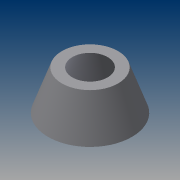
# Autodesk Inventor part: pin
Saved by Autodesk Inventor 2020 (Build 240168000, 168)
## iProperties
Created: 2021-10-08
Part Number: pin
Material: Genérico
Document SubType Name: Modeling
Designer: MATT
Density: 1 g/cm^3
Appearance: Por defecto
Mass: 0.101116 g
Surface Area: 8.28121 cm^2
Volume: 0.101116 cm^3
Author: MATT
Autodesk Inventor part; units mm, degrees
ref_plane "YZ Plane" through (0, 0, 0) normal (1, 0, 0) x (0, 1, 0)
ref_plane "XZ Plane" through (0, 0, 0) normal (0, 1, 0) x (-1, 0, 0)
ref_plane "XY Plane" through (0, 0, 0) normal (0, 0, 1) x (1, 0, 0)
sketch "Boceto1" plane through (0, 0, 0) normal (0, 1, 0) x (-1, 0, 0)
  circle A0 centre (0, 0) radius 7.5
  circle A1 centre (0, 0) radius 8.5
  dimension "d0" = 15
  dimension "d14" = 17
  constraints: 2 centre point, 2 coincident
  measures "d0" diameter of A0
  measures "d14" diameter of A1
sketch "Boceto2" plane through (0, 0, 0) normal (1, 0, 0) x (0, 1, 0)
  line L0 (0, 0) -> (10, 0)
  dimension "d1" = 10
  constraints: 2 end point, 1 horizontal
  measures "d1" distance of L0.start L0.end
ref_plane "Work Plane3" through (0, 10, 0) normal (0, 1, 0) x (-1, 0, 0)
ref_plane "Plano de trabajo1" through (0, 10, 0) normal (0, 1, 0) x (-1, 0, 0)
sketch "Sketch6" plane through (0, 10, 0) normal (0, 1, 0) x (-1, 0, 0)
  circle A0 centre (0, 0) radius 5
  circle A1 centre (0, 0) radius 6
  dimension "d12" = 10
  dimension "d13" = 12
  constraints: 2 centre point, 2 coincident
  measures "d12" diameter of A0
  measures "d13" diameter of A1
loft "Loft2" add profiles "Sketch6", "Boceto1" contours A0 / A0 | A1
shell "Shell2" thickness 2 removed faces 1 at (3.0201, 0, -2.8939)
shell "Shell3" thickness 2 removed faces 3 at (0.591, 10, 1.5584) at (-7.4978, 2.2222, -1.848) at (-0.6057, 8, 0.7916)
body "Solid2"
